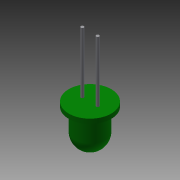
# Autodesk Inventor part: licht_led_gruen
Saved by Autodesk Inventor 2015 (Build 190159000, 159)
## iProperties
Created: 2018-01-12
Part Number: licht_led_gruen
Material: Generisch
Document SubType Name: Modeling
Designer: wepet
Density: 1 g/cm^3
Appearance: Vorgabe
Author: wepet
Autodesk Inventor part; units mm, degrees
ref_plane "YZ Plane" through (0, 0, 0) normal (1, 0, 0) x (0, 1, 0)
ref_plane "XZ Plane" through (0, 0, 0) normal (0, 1, 0) x (-1, 0, 0)
ref_plane "XY Plane" through (0, 0, 0) normal (0, 0, 1) x (1, 0, 0)
sketch "Skizze1" plane through (0, 0, 0) normal (0, 1, 0) x (-1, 0, 0)
  line L0 (0, 0) -> (3.5, 0)
  line L1 (3.5, 0) -> (3.5, -0.75)
  line L2 (3.5, -0.75) -> (2.5, -0.75)
  line L3 (2.5, -0.75) -> (2.5, -4.25)
  line L4 (0, -6.75) -> (0, -6.75)
  line L5 (0, -6.75) -> (0, 0)
  arc A0 (0, -6.75) -> (2.5, -4.25) centre (0, -4.25) ccw
  point P0 (2.5, -6.75)
  dimension "d6" = 3.5
  dimension "d7" = 0.75
  dimension "d8" = 1
  dimension "d9" = 6
  dimension "d10" = 2.5
  constraints: 12 end point, 5 perpendicular, 2 point on circle, 2 point on line, 2 tangent, 1 centre point, 1 coincident, 1 horizontal
  measures "d6" distance of L0.start L0.end
  measures "d7" distance of L0.end L1.end
  measures "d8" distance of L1.end L2.end
  measures "d9" distance of L2.end point (2.5, -6.75)
  measures "d10" radius of A0
revolve "Umdrehung1" add sketch "Skizze1" angle 360 about axis through (0, 0, -6.75) along (0, 0, 1)
sketch "Skizze2" plane through (0, 0, 0) normal (0, 0, 1) x (1, 0, 0)
  circle A0 centre (0, 0) radius 3.5 projected
  circle A1 centre (0, 0) radius 3.5 projected
  circle A2 centre (-1.27, 0) radius 0.25
  circle A3 centre (1.27, 0) radius 0.25
  point P0 (0, 0)
  dimension "d11" = 0.5
  dimension "d12" = 0.5
  dimension "d13" = 1.27
  dimension "d14" = 1.27
  constraints: 2 centre point
  measures "d11" diameter of A2
  measures "d12" diameter of A3
  measures "d13" distance of A3.centre point (0, 0)
  measures "d14" distance of A2.centre point (0, 0)
extrude "Extrusion1" add sketch "Skizze2" along normal blind 10 contours A2 | A3
